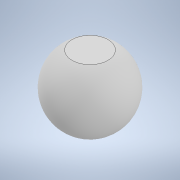
# Autodesk Inventor part: Ball
Saved by Autodesk Inventor 2022 (Build 260153000, 153)
## iProperties
Created: 2022-08-27
Part Number: Ball
Material: Generic
Document SubType Name: Modeling
Designer: Nick
Density: 1 g/cm^3
Appearance: Default
Author: Nick
Autodesk Inventor part; units mm, degrees
ref_plane "YZ Plane" through (0, 0, 0) normal (1, 0, 0) x (0, 1, 0)
ref_plane "XZ Plane" through (0, 0, 0) normal (0, 1, 0) x (-1, 0, 0)
ref_plane "XY Plane" through (0, 0, 0) normal (0, 0, 1) x (1, 0, 0)
sketch "Sketch1" plane through (0, 0, 0) normal (0, 0, 1) x (1, 0, 0)
  circle A0 centre (0, 0) radius 5
  line L0 (-3.2169, -5) -> (4.2904, -5) construction
  line L1 (-2.4296, 4.37) -> (2.4296, 4.37)
  line L2 (0, 4.37) -> (0, -5)
  dimension "d0" = 10
  dimension "d1" = 9.37
  constraints: 6 end point, 3 point on circle, 2 horizontal, 1 centre point, 1 coincident, 1 midpoint, 1 point on line, 1 tangent
  measures "d0" diameter of A0
  measures "d1" distance between parallel lines of L1 L0
revolve "Revolution1" add sketch "Sketch1" angle 360 about axis through (0, 4.37, 0) along (0, -1, 0) picked at (-0.3953, -1.8291) contours A0 L1 L2
body "Solid1"
